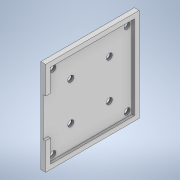
# Autodesk Inventor part: Mag_Shield_Back
Saved by Autodesk Inventor 2022 (Build 260153000, 153)
## iProperties
Created: 2022-03-10
Part Number: Mag_Shield_Back
Material: Generic
Document SubType Name: Modeling
Designer: Mlees
Density: 1 g/cm^3
Appearance: Default
Author: Mlees
Autodesk Inventor part; units mm, degrees
ref_plane "YZ Plane" through (0, 0, 0) normal (1, 0, 0) x (0, 1, 0)
ref_plane "XZ Plane" through (0, 0, 0) normal (0, 1, 0) x (-1, 0, 0)
ref_plane "XY Plane" through (0, 0, 0) normal (0, 0, 1) x (1, 0, 0)
sketch "Sketch1" plane through (0, 0, 0) normal (1, 0, 0) x (0, 1, 0)
  line L0 (0, 0) -> (30.75, 0)
  line L1 (30.75, 0) -> (30.75, -30.75)
  line L2 (30.75, -30.75) -> (0, -30.75)
  line L3 (0, -30.75) -> (0, 0)
  line L4 (32.75, -32.75) -> (32.75, 2)
  line L5 (32.75, 2) -> (-2, 2)
  line L6 (-2, 2) -> (-2, -32.75)
  line L7 (-2, -32.75) -> (32.75, -32.75)
  circle A0 centre (30.75, 0) radius 1.25
  circle A1 centre (30.75, -30.75) radius 1.25
  circle A2 centre (0, -30.75) radius 1.25
  circle A3 centre (0, 0) radius 1.25
  line L8 (-4, 4) -> (34.75, 4)
  line L9 (34.75, 4) -> (34.75, -34.75)
  line L10 (34.75, -34.75) -> (-4, -34.75)
  line L11 (-4, -34.75) -> (-4, 4)
  circle A4 centre (7.375, -7.375) radius 1.25
  circle A5 centre (7.375, -23.375) radius 1.25
  circle A6 centre (23.375, -23.375) radius 1.25
  circle A7 centre (23.375, -7.375) radius 1.25
  dimension "d0" = 30.75
  dimension "d1" = 30.75
  dimension "d2" = 2
  dimension "d3" = 2.5
  dimension "d4" = 2
  dimension "d14" = 2.5
  constraints: 24 end point, 8 centre point, 6 parallel, 4 coincident, 3 perpendicular, 1 horizontal, 6 other
  measures "d0" distance of L1.end L2.end
  measures "d1" distance of L0.end L1.end
  measures "d2" distance between parallel lines of L1 L4
  measures "d3" diameter of A0
  measures "d4" distance between parallel lines of L5 L8
  measures "d14" diameter of A4
extrude "Extrusion3" add sketch "Sketch1" along normal blind 1 contours L0 A0 L1 A1 L2 A2 L3 A3 | L7 L6 L5 L4 | L8 L9 L10 L11
sketch "Sketch3" plane through (1, 0, 0) normal (1, 0, 0) x (0, 0, -1)
  line L0 (-4, -4) -> (34.75, -4) projected
  line L1 (34.75, -4) -> (34.75, 34.75) projected
  line L2 (-4, -4) -> (34.75, -4)
  line L3 (34.75, -4) -> (34.75, 34.75)
  line L4 (34.75, 34.75) -> (-4, 34.75)
  line L5 (-4, 34.75) -> (-4, -4)
  line L6 (-2, -2) -> (32.75, -2)
  line L7 (32.75, -2) -> (32.75, 32.75)
  line L8 (32.75, 32.75) -> (-2, 32.75)
  line L9 (-2, 32.75) -> (-2, -2)
  point P0 (0, 0)
  dimension "d17" = 2
  constraints: 16 end point, 4 parallel, 2 perpendicular, 1 horizontal, 3 other
  measures "d17" distance between parallel lines of L5 L9
extrude "Extrusion4" add sketch "Sketch3" along normal blind 1
sketch "Sketch4" plane through (2, 0, 0) normal (1, 0, 0) x (0, 0, -1)
  line L0 (-2, 32.75) -> (-2, -2) projected
  line L1 (-2, 15.375) -> (-2, 23.375)
  line L2 (-2, 23.375) -> (-4, 23.375)
  line L3 (-4, 34.75) -> (-4, -4) projected
  line L4 (-4, 23.375) -> (-4, 7.375)
  line L5 (-4, 7.375) -> (-2, 7.375)
  line L6 (-2, 7.375) -> (-2, 15.375)
  point P0 (0, 0)
  dimension "d20" = 8
  dimension "d21" = 16
  constraints: 10 end point, 3 perpendicular, 3 point on line, 1 midpoint, 1 parallel
  measures "d20" distance of L1.start L1.end
  measures "d21" distance of L2.end L4.end
extrude "Extrusion5" cut sketch "Sketch4" against normal blind 1
body "Solid2"
